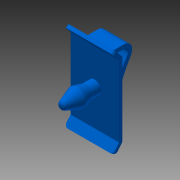
# Autodesk Inventor part: W116_Clip_Inv
Saved by Autodesk Inventor 2014 SP2 (Build 180246200, 246)
## iProperties
Created: 2014-07-31
Part Number: W116_Clip_Inv
Material: PLA Plastic
Document SubType Name: Modeling
Designer: Lukasz Szmit
Density: 1.21 g/cm^3
Appearance: Generic
Author: Lukasz Szmit
Autodesk Inventor part; units mm, degrees
ref_plane "YZ Plane" through (0, 0, 0) normal (1, 0, 0) x (0, 1, 0)
ref_plane "XZ Plane" through (0, 0, 0) normal (0, 1, 0) x (-1, 0, 0)
ref_plane "XY Plane" through (0, 0, 0) normal (0, 0, 1) x (1, 0, 0)
sketch "Base" plane through (0, 0, 0) normal (0, 1, 0) x (-1, 0, 0)
  line L0 (-7.375, -10.7) -> (-7.375, 10.7)
  line L1 (7.375, 10.7) -> (7.375, 13.5)
  line L2 (6.375, 14.5) -> (-6.375, 14.5)
  line L3 (-7.375, 13.5) -> (-7.375, 10.7)
  line L4 (7.375, -10.7) -> (7.375, -13.5)
  line L5 (6.375, -14.5) -> (-6.375, -14.5)
  line L6 (-7.375, -13.5) -> (-7.375, -10.7)
  line L7 (7.375, 10.7) -> (7.375, -10.7)
  arc A0 (-6.375, 14.5) -> (-7.375, 13.5) centre (-6.375, 13.5) ccw
  arc A1 (7.375, 13.5) -> (6.375, 14.5) centre (6.375, 13.5) ccw
  arc A2 (6.375, -14.5) -> (7.375, -13.5) centre (6.375, -13.5) ccw
  arc A3 (-7.375, -13.5) -> (-6.375, -14.5) centre (-6.375, -13.5) ccw
  point P0 (0, 0)
  point P1 (7.375, 14.5)
  point P2 (-7.375, 14.5)
  point P3 (7.375, -14.5)
  point P4 (-7.375, -14.5)
  dimension "d114" = 90
  dimension "d115" = 90
  dimension "d118" = 29
  dimension "d119" = 7.375
  dimension "d120" = 14.5
  dimension "d122" = 3.8
  dimension "d124" = 25.2
  dimension "d125" = 3.8
  dimension "d126" = 25.2
  dimension "d127" = 14.75
  dimension "d215" = 1
  constraints: 16 end point, 8 point on circle, 8 point on line, 8 tangent, 4 centre point, 3 equal radius, 3 parallel, 2 vertical, 1 horizontal
  measures "d114" angle of L1 L2
  measures "d115" angle of L2 L3
  measures "d118" distance between parallel lines of L2 L5
  measures "d119" distance from line of point (0, 0) L1
  measures "d120" distance from line of point (0, 0) L2
  measures "d122" distance from line of L1.start L2
  measures "d124" distance from line of L4.start L2
  measures "d125" distance from line of L0.end L2
  measures "d126" distance from line of L0.start L2
  measures "d127" distance between parallel lines of L7 L3
  measures "d215" radius of A0
sketch "Support" plane through (0, 0, 0) normal (1, 0, 0) x (0, 1, 0)
  arc A0 (6.3903, 8.3286) -> (3.8899, 10.8289) centre (3.8901, 8.3286) ccw
  line L0 (6.3903, 8.3286) -> (6.3903, 5.7644) construction
  spline S0 degree 3 poles (6.3903, 8.3286) (6.3903, 5.7644) (3.3686, 5.7643) (0, -10.5713) knots 1 1 1 1 1.99994 1.99994 1.99994 1.99994
  line L1 (3.8899, 10.8289) -> (0, 10.8287)
  line L2 (6.3903, 5.7644) -> (3.3686, 5.7643) construction
  line L3 (3.3686, 5.7643) -> (0, -10.5713) construction
  line L4 (0, 10.8287) -> (0, -10.5713)
  point P0 (0, 0)
  point P1 (-0.0055, 6.3833)
  dimension "d202" = 2.5003
  dimension "d203" = 11.652
  dimension "d204" = 6.3903
  dimension "d205" = 5.7641
  dimension "d206" = 2.4416
  dimension "d207" = 3.0218
  dimension "d208" = 6.3903
  dimension "d209" = 6.3958
  dimension "d210" = 0.6192
  dimension "d211" = 21.4
  constraints: 4 end point, 2 parallel, 2 point on circle, 2 tangent, 1 centre point, 1 vertical, 4 other
  measures "d202" radius of A0
  measures "d203" angle of L3 L4
  measures "d204" distance from line of point (0, 0) L0
  measures "d205" distance from line of point (0, 0) L2
  measures "d206" distance from line of L0.start L3
  measures "d207" distance from line of L2.end L0
  measures "d208" distance from line of L1.end L0
  measures "d209" distance from line of point (-0.005, 6.383) L0
  measures "d210" distance from line of point (-0.005, 6.383) L2
  measures "d211" distance of L3.end L1.end
sketch "Shaft" plane through (0, 0, 0) normal (0, 0, 1) x (1, 0, 0)
  line L0 (1.933, -1) -> (1.933, -3.5)
  line L1 (-0.067, -11.3406) -> (0.2327, -11.3406)
  line L2 (1.933, -3.5) -> (2.6374, -6.1289)
  line L3 (2.6111, -6.7298) -> (1.1724, -10.6826)
  arc A0 (0.2327, -11.3406) -> (1.1724, -10.6826) centre (0.2327, -10.3406) ccw
  line L4 (-0.067, -1) -> (-0.067, -11.3406)
  line L5 (-0.067, -1) -> (1.933, -1)
  arc A1 (2.6111, -6.7298) -> (2.6374, -6.1289) centre (1.6714, -6.3878) ccw
  point P0 (0, 0)
  point P1 (0.933, -11.3406)
  point P2 (-0.3499, -10.7665)
  point P3 (2.6305, -6.6765)
  point P4 (2.6142, -6.0424)
  point P5 (0, 0)
  point P6 (0, 0)
  dimension "d57" = 2.5
  dimension "d58" = 1
  dimension "d59" = 0.64
  dimension "d61" = 2
  dimension "d62" = 1
  dimension "d63" = 165
  dimension "d64" = 145
  dimension "d65" = 10.3406
  dimension "d66" = 0.9612
  dimension "d67" = 4.0858
  dimension "d148" = 1
  dimension "d149" = 0.1483
  dimension "d150" = 0.6812
  constraints: 12 end point, 4 point on circle, 4 point on line, 4 tangent, 2 centre point, 2 coincident, 1 equal radius, 1 horizontal, 1 parallel, 1 perpendicular
  measures "d57" distance of L5.end L0.end
  measures "d58" distance of L4.end point (0.933, -11.341)
  measures "d59" distance of L4.end point (-0.35, -10.766)
  measures "d61" distance between parallel lines of L4 L0
  measures "d62" vertical distance of point (0, 0) L5.start
  measures "d63" angle of L2 L0
  measures "d64" angle of L3 L2
  measures "d65" distance between parallel lines of L1 L5
  measures "d66" distance from line of point (0, 0) L2
  measures "d67" distance from line of point (-0.35, -10.766) L2
  measures "d148" radius of A1
  measures "d149" distance from line of point (2.631, -6.677) L2
  measures "d150" distance from line of point (2.614, -6.042) L0
extrude "Base Extrusion" add sketch "Base" against normal blind 1
sketch "Sketch4" plane through (0, 0, 0) normal (0, 1, 0) x (-1, 0, 0)
  line L0 (10.6853, -10.7) -> (-11.8595, -10.7)
  line L1 (12.5464, 10.7) -> (-12.5363, 10.7)
  line L2 (6.375, 14.5) -> (-6.375, 14.5) projected
  line L3 (-6.375, -14.5) -> (6.375, -14.5) projected
  point P0 (0, 0)
  point P1 (7.375, 14.5)
  point P2 (-7.375, 14.5)
  point P3 (-7.375, -14.5)
  point P4 (7.375, -14.5)
  dimension "d130" = 3.8
  dimension "d131" = 3.8
  constraints: 4 end point
  measures "d130" distance between parallel lines of L1 L2
  measures "d131" distance between parallel lines of L3 L0
bend part "Base Bend 1" radius 1.4324 angle 40 line through (-10.6853, 0, -10.7) along (1, 0, 0) centre toward (0, -1, 0) moving side (0, 0, -1) both sides no
sketch "Sketch5" plane through (0, 0, 0) normal (0, 1, 0) x (1, 0, 0)
  line L0 (-6.375, -14.5) -> (6.375, -14.5) projected
  line L1 (-11.4458, -10.7) -> (11.7638, -10.7)
  point P0 (-7.375, -14.5)
  point P1 (7.375, -14.5)
  point P2 (0, 0)
  dimension "d134" = 3.8
  constraints: 2 end point
  measures "d134" distance between parallel lines of L0 L1
bend part "Base Bend 2" radius 1.4324 angle 40 line through (-11.4458, 0, 10.7) along (1, 0, 0) centre toward (0, -1, 0) moving side (0, 0, 1) both sides no
revolve "Shaft Solid" add sketch "Shaft" angle 360 about axis through (-0.067, -1, 0) along (0, -1, 0)
extrude "Extrusion11" add sketch "Support" along normal blind 3.95 and the other way blind 3.95
sketch "Sketch11" plane through (3.95, 0, 0) normal (1, 0, 0) x (0, 0, -1)
  arc A0 (-8.3286, 6.3903) -> (-10.8289, 3.8899) centre (-8.3286, 3.8901) ccw projected
  line L0 (10.5713, 0) -> (-10.7, 0) projected
  spline S0 degree 3 poles (10.5713, 0) (-5.7643, 3.3686) (-5.7644, 6.3903) (-8.3286, 6.3903) knots 0 0 0 0 1 1 1 1
  arc A1 (-8.3286, 5.1403) -> (-9.5789, 3.89) centre (-8.3286, 3.8901) ccw
  line L1 (-9.5789, 3.89) -> (-9.5789, 0)
  line L2 (-9.5789, 0) -> (-1.5789, 0)
  line L3 (-1.5789, 0) -> (-1.5789, 2.0292)
  spline S1 degree 5 poles (-1.5789, 2.0292) (-1.8424, 2.1293) (-2.1051, 2.2316) (-2.3668, 2.3364) (-3.2454, 2.6977) (-4.1111, 3.0893) (-4.7126, 3.3815) (-5.6283, 3.8657) (-6.5238, 4.3869) (-6.8409, 4.5714) (-7.3068, 4.8546) (-7.8075, 5.0665) (-7.9761, 5.1228) (-8.1536, 5.1402) (-8.3286, 5.1403) knots 0 0 0 0 0 0 0.188799 0.188799 0.188799 0.636245 0.636245 0.636245 0.882484 0.882484 0.882484 1 1 1 1 1 1
  point P0 (0, 0)
  constraints: 6 end point, 3 point on line, 2 point on circle, 1 centre point, 7 other
extrude "Extrusion12" cut sketch "Sketch11" against normal blind 7.9
body "Solid3"
